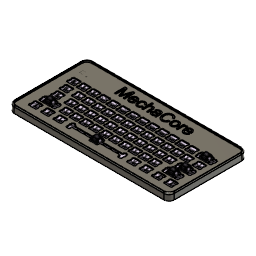
Mechacore (Autodesk Fusion 360 design; units mm, degrees)
description: KiCad electronic assembly
part number: Mechacore 1
part number: D_SOD-123
part number: SW_Cherry_MX_PCB
Autodesk Fusion 360 part; units mm, degrees
(part 1 of 4)
sketch "Sketch1" plane through (0, 0, 0) normal (0, 1, 0) x (1, 0, 0)
  line L0 (0, 0) -> (310, 0)
  line L1 (310, 0) -> (310, 150.9928)
  line L2 (310, 150.9928) -> (0, 150.9928)
  line L3 (0, 150.9928) -> (0, 0)
  dimension "d1" = 310
  constraint horizontal L0
  constraint vertical L1
  constraint horizontal L2
  constraint vertical L3
  constraint coincident L0.start L3.end
  measures "d1" distance of L0.start L0.end
extrude "Extrude1" add sketch "Sketch1" along normal blind 10 makes body 1
extrude "Extrude2" add 1 faces at (206.6667, 10, -50.3309) along direction (0, 1, 0) blind 4 on bodies 1 bodies 1
shell "Shell1" thickness 2 removed faces 1 at (206.6667, 14, -50.3309) on bodies 1
fillet "Fillet1" radius 10 1 edges at (2, 8, -148.9928) on bodies 1
fillet "Fillet2" radius 10 1 edges at (308, 8, -148.9928) on bodies 1
fillet "Fillet3" radius 10 1 edges at (308, 8, -2) on bodies 1
fillet "Fillet4" radius 10 1 edges at (2, 8, -2) on bodies 1
fillet "Fillet5" radius 10 3 edges at (310, 7, -150.9928) (0, 7, -150.9928) (310, 7, 0) on bodies 1
fillet "Fillet6" radius 10 1 edges at (0, 7, 0) on bodies 1
other "Base Mesh Feature1"
other "Modify1"
other "Modify2"
sketch "48cd8e48e3c34c88b59e201f8eb7611360cf066c_switch" plane through (0, 0, 0) normal (0, 1, 0) x (1, 0, 0)
  line L0 (0.0951, 95.5075) -> (285.845, 95.5075)
  line L1 (285.845, 95.5075) -> (285.845, 0.2577)
  line L2 (285.845, 0.2577) -> (0.0951, 0.2577)
  line L3 (0.0951, 0.2577) -> (0.0951, 95.5075)
  line L4 (124.062, 16.7831) -> (124.062, 15.7827)
  line L5 (124.062, 15.7827) -> (123.263, 15.7827)
  line L6 (123.263, 15.7827) -> (123.263, 12.6848)
  line L7 (123.263, 12.6848) -> (124.062, 12.6848)
  line L8 (124.062, 12.6848) -> (124.062, 12.0826)
  line L9 (124.062, 12.0826) -> (84.4381, 12.0826)
  line L10 (84.4381, 12.0826) -> (84.4381, 15.3128)
  line L11 (84.4381, 15.3128) -> (82.7126, 15.3128)
  line L12 (82.7126, 15.3128) -> (82.7126, 16.2347)
  line L13 (82.7126, 16.2347) -> (79.412, 16.2347)
  line L14 (79.412, 16.2347) -> (79.412, 15.3128)
  line L15 (79.412, 15.3128) -> (77.687, 15.3128)
  line L16 (77.687, 15.3128) -> (77.687, 12.0826)
  line L17 (77.687, 12.0826) -> (76.8629, 12.0826)
  line L18 (76.8629, 12.0826) -> (76.8629, 9.2838)
  line L19 (76.8629, 9.2838) -> (77.687, 9.2838)
  line L20 (77.687, 9.2838) -> (77.687, 3.0138)
  line L21 (77.687, 3.0138) -> (79.412, 3.0138)
  line L22 (79.412, 3.0138) -> (79.412, 2.0326)
  line L23 (79.412, 2.0326) -> (82.7126, 2.0326)
  line L24 (82.7126, 2.0326) -> (82.7126, 3.0138)
  line L25 (82.7126, 3.0138) -> (84.4381, 3.0138)
  line L26 (84.4381, 3.0138) -> (84.4381, 7.4841)
  line L27 (84.4381, 7.4841) -> (124.062, 7.4841)
  line L28 (124.062, 7.4841) -> (124.062, 6.8833)
  line L29 (124.062, 6.8833) -> (123.263, 6.8833)
  line L30 (123.263, 6.8833) -> (123.263, 3.7827)
  line L31 (123.263, 3.7827) -> (124.062, 3.7827)
  line L32 (124.062, 3.7827) -> (124.062, 2.7836)
  line L33 (124.062, 2.7836) -> (138.063, 2.7836)
  line L34 (138.063, 2.7836) -> (138.063, 3.7827)
  line L35 (138.063, 3.7827) -> (138.862, 3.7827)
  line L36 (138.862, 3.7827) -> (138.862, 6.8833)
  line L37 (138.862, 6.8833) -> (138.063, 6.8833)
  line L38 (138.063, 6.8833) -> (138.063, 7.4841)
  line L39 (138.063, 7.4841) -> (177.687, 7.4841)
  line L40 (177.687, 7.4841) -> (177.687, 3.0138)
  line L41 (177.687, 3.0138) -> (179.412, 3.0138)
  line L42 (179.412, 3.0138) -> (179.412, 2.0326)
  line L43 (179.412, 2.0326) -> (182.713, 2.0326)
  line L44 (182.713, 2.0326) -> (182.713, 3.0138)
  line L45 (182.713, 3.0138) -> (184.438, 3.0138)
  line L46 (184.438, 3.0138) -> (184.438, 9.2838)
  line L47 (184.438, 9.2838) -> (185.262, 9.2838)
  line L48 (185.262, 9.2838) -> (185.262, 12.0826)
  line L49 (185.262, 12.0826) -> (184.438, 12.0826)
  line L50 (184.438, 12.0826) -> (184.438, 15.3128)
  line L51 (184.438, 15.3128) -> (182.713, 15.3128)
  line L52 (182.713, 15.3128) -> (182.713, 16.2347)
  line L53 (182.713, 16.2347) -> (179.412, 16.2347)
  line L54 (179.412, 16.2347) -> (179.412, 15.3128)
  line L55 (179.412, 15.3128) -> (177.687, 15.3128)
  line L56 (177.687, 15.3128) -> (177.687, 12.0826)
  line L57 (177.687, 12.0826) -> (138.063, 12.0826)
  line L58 (138.063, 12.0826) -> (138.063, 12.6848)
  line L59 (138.063, 12.6848) -> (138.862, 12.6848)
  line L60 (138.862, 12.6848) -> (138.862, 15.7827)
  line L61 (138.862, 15.7827) -> (138.063, 15.7827)
  line L62 (138.063, 15.7827) -> (138.063, 16.7831)
  line L63 (138.063, 16.7831) -> (124.062, 16.7831)
  line L64 (5.0009, 16.7831) -> (5.0009, 15.7827)
  line L65 (5.0009, 15.7827) -> (4.2003, 15.7827)
  line L66 (4.2003, 15.7827) -> (4.2003, 12.6848)
  line L67 (4.2003, 12.6848) -> (5.0009, 12.6848)
  line L68 (5.0009, 12.6848) -> (5.0009, 6.8833)
  line L69 (5.0009, 6.8833) -> (4.2003, 6.8833)
  line L70 (4.2003, 6.8833) -> (4.2003, 3.7827)
  line L71 (4.2003, 3.7827) -> (5.0009, 3.7827)
  line L72 (5.0009, 3.7827) -> (5.0009, 2.7836)
  line L73 (5.0009, 2.7836) -> (19.0004, 2.7836)
  line L74 (19.0004, 2.7836) -> (19.0004, 3.7827)
  line L75 (19.0004, 3.7827) -> (19.801, 3.7827)
  line L76 (19.801, 3.7827) -> (19.801, 6.8833)
  line L77 (19.801, 6.8833) -> (19.0004, 6.8833)
  line L78 (19.0004, 6.8833) -> (19.0004, 12.6848)
  line L79 (19.0004, 12.6848) -> (19.801, 12.6848)
  line L80 (19.801, 12.6848) -> (19.801, 15.7827)
  line L81 (19.801, 15.7827) -> (19.0004, 15.7827)
  line L82 (19.0004, 15.7827) -> (19.0004, 16.7831)
  line L83 (19.0004, 16.7831) -> (5.0009, 16.7831)
  line L84 (28.812, 16.7831) -> (28.812, 15.7827)
  line L85 (28.812, 15.7827) -> (28.0128, 15.7827)
  line L86 (28.0128, 15.7827) -> (28.0128, 12.6848)
  line L87 (28.0128, 12.6848) -> (28.812, 12.6848)
  line L88 (28.812, 12.6848) -> (28.812, 6.8833)
  line L89 (28.812, 6.8833) -> (28.0128, 6.8833)
  line L90 (28.0128, 6.8833) -> (28.0128, 3.7827)
  line L91 (28.0128, 3.7827) -> (28.812, 3.7827)
  line L92 (28.812, 3.7827) -> (28.812, 2.7836)
  line L93 (28.812, 2.7836) -> (42.8128, 2.7836)
  line L94 (42.8128, 2.7836) -> (42.8128, 3.7827)
  line L95 (42.8128, 3.7827) -> (43.6122, 3.7827)
  line L96 (43.6122, 3.7827) -> (43.6122, 6.8833)
  line L97 (43.6122, 6.8833) -> (42.8128, 6.8833)
  line L98 (42.8128, 6.8833) -> (42.8128, 12.6848)
  line L99 (42.8128, 12.6848) -> (43.6122, 12.6848)
  line L100 (43.6122, 12.6848) -> (43.6122, 15.7827)
  line L101 (43.6122, 15.7827) -> (42.8128, 15.7827)
  line L102 (42.8128, 15.7827) -> (42.8128, 16.7831)
  line L103 (42.8128, 16.7831) -> (28.812, 16.7831)
  line L104 (52.626, 16.7831) -> (52.626, 15.7827)
  line L105 (52.626, 15.7827) -> (51.8252, 15.7827)
  line L106 (51.8252, 15.7827) -> (51.8252, 12.6848)
  line L107 (51.8252, 12.6848) -> (52.626, 12.6848)
  line L108 (52.626, 12.6848) -> (52.626, 6.8833)
  line L109 (52.626, 6.8833) -> (51.8252, 6.8833)
  line L110 (51.8252, 6.8833) -> (51.8252, 3.7827)
  line L111 (51.8252, 3.7827) -> (52.626, 3.7827)
  line L112 (52.626, 3.7827) -> (52.626, 2.7836)
  line L113 (52.626, 2.7836) -> (66.6253, 2.7836)
  line L114 (66.6253, 2.7836) -> (66.6253, 3.7827)
  line L115 (66.6253, 3.7827) -> (67.4261, 3.7827)
  line L116 (67.4261, 3.7827) -> (67.4261, 6.8833)
  line L117 (67.4261, 6.8833) -> (66.6253, 6.8833)
  line L118 (66.6253, 6.8833) -> (66.6253, 12.6848)
  line L119 (66.6253, 12.6848) -> (67.4261, 12.6848)
  line L120 (67.4261, 12.6848) -> (67.4261, 15.7827)
  line L121 (67.4261, 15.7827) -> (66.6253, 15.7827)
  line L122 (66.6253, 15.7827) -> (66.6253, 16.7831)
  line L123 (66.6253, 16.7831) -> (52.626, 16.7831)
  line L124 (195.501, 16.7831) -> (195.501, 15.7827)
  line L125 (195.501, 15.7827) -> (194.7, 15.7827)
  line L126 (194.7, 15.7827) -> (194.7, 12.6848)
  line L127 (194.7, 12.6848) -> (195.501, 12.6848)
  line L128 (195.501, 12.6848) -> (195.501, 6.8833)
  line L129 (195.501, 6.8833) -> (194.7, 6.8833)
  line L130 (194.7, 6.8833) -> (194.7, 3.7827)
  line L131 (194.7, 3.7827) -> (195.501, 3.7827)
  line L132 (195.501, 3.7827) -> (195.501, 2.7836)
  line L133 (195.501, 2.7836) -> (209.5, 2.7836)
  line L134 (209.5, 2.7836) -> (209.5, 3.7827)
  line L135 (209.5, 3.7827) -> (210.301, 3.7827)
  line L136 (210.301, 3.7827) -> (210.301, 6.8833)
  line L137 (210.301, 6.8833) -> (209.5, 6.8833)
  line L138 (209.5, 6.8833) -> (209.5, 12.6848)
  line L139 (209.5, 12.6848) -> (210.301, 12.6848)
  line L140 (210.301, 12.6848) -> (210.301, 15.7827)
  line L141 (210.301, 15.7827) -> (209.5, 15.7827)
  line L142 (209.5, 15.7827) -> (209.5, 16.7831)
  line L143 (209.5, 16.7831) -> (195.501, 16.7831)
  line L144 (219.312, 16.7831) -> (219.312, 15.7827)
  line L145 (219.312, 15.7827) -> (218.513, 15.7827)
  line L146 (218.513, 15.7827) -> (218.513, 12.6848)
  line L147 (218.513, 12.6848) -> (219.312, 12.6848)
  line L148 (219.312, 12.6848) -> (219.312, 6.8833)
  line L149 (219.312, 6.8833) -> (218.513, 6.8833)
  line L150 (218.513, 6.8833) -> (218.513, 3.7827)
  line L151 (218.513, 3.7827) -> (219.312, 3.7827)
  line L152 (219.312, 3.7827) -> (219.312, 2.7836)
  line L153 (219.312, 2.7836) -> (233.313, 2.7836)
  line L154 (233.313, 2.7836) -> (233.313, 3.7827)
  line L155 (233.313, 3.7827) -> (234.112, 3.7827)
  line L156 (234.112, 3.7827) -> (234.112, 6.8833)
  line L157 (234.112, 6.8833) -> (233.313, 6.8833)
  line L158 (233.313, 6.8833) -> (233.313, 12.6848)
  line L159 (233.313, 12.6848) -> (234.112, 12.6848)
  line L160 (234.112, 12.6848) -> (234.112, 15.7827)
  line L161 (234.112, 15.7827) -> (233.313, 15.7827)
  line L162 (233.313, 15.7827) -> (233.313, 16.7831)
  line L163 (233.313, 16.7831) -> (219.312, 16.7831)
  line L164 (243.126, 16.7831) -> (243.126, 15.7827)
  line L165 (243.126, 15.7827) -> (242.325, 15.7827)
  line L166 (242.325, 15.7827) -> (242.325, 12.6848)
  line L167 (242.325, 12.6848) -> (243.126, 12.6848)
  line L168 (243.126, 12.6848) -> (243.126, 6.8833)
  line L169 (243.126, 6.8833) -> (242.325, 6.8833)
  line L170 (242.325, 6.8833) -> (242.325, 3.7827)
  line L171 (242.325, 3.7827) -> (243.126, 3.7827)
  line L172 (243.126, 3.7827) -> (243.126, 2.7836)
  line L173 (243.126, 2.7836) -> (257.125, 2.7836)
  line L174 (257.125, 2.7836) -> (257.125, 3.7827)
  line L175 (257.125, 3.7827) -> (257.926, 3.7827)
  line L176 (257.926, 3.7827) -> (257.926, 6.8833)
  line L177 (257.926, 6.8833) -> (257.125, 6.8833)
  line L178 (257.125, 6.8833) -> (257.125, 12.6848)
  line L179 (257.125, 12.6848) -> (257.926, 12.6848)
  line L180 (257.926, 12.6848) -> (257.926, 15.7827)
  line L181 (257.926, 15.7827) -> (257.125, 15.7827)
  line L182 (257.125, 15.7827) -> (257.125, 16.7831)
  line L183 (257.125, 16.7831) -> (243.126, 16.7831)
  line L184 (266.937, 16.7831) -> (266.937, 15.7827)
  line L185 (266.937, 15.7827) -> (266.138, 15.7827)
  line L186 (266.138, 15.7827) -> (266.138, 12.6848)
  line L187 (266.138, 12.6848) -> (266.937, 12.6848)
  line L188 (266.937, 12.6848) -> (266.937, 6.8833)
  line L189 (266.937, 6.8833) -> (266.138, 6.8833)
  line L190 (266.138, 6.8833) -> (266.138, 3.7827)
  line L191 (266.138, 3.7827) -> (266.937, 3.7827)
  line L192 (266.937, 3.7827) -> (266.937, 2.7836)
  line L193 (266.937, 2.7836) -> (280.938, 2.7836)
  line L194 (280.938, 2.7836) -> (280.938, 3.7827)
  line L195 (280.938, 3.7827) -> (281.737, 3.7827)
  line L196 (281.737, 3.7827) -> (281.737, 6.8833)
  line L197 (281.737, 6.8833) -> (280.938, 6.8833)
  line L198 (280.938, 6.8833) -> (280.938, 12.6848)
  line L199 (280.938, 12.6848) -> (281.737, 12.6848)
  line L200 (281.737, 12.6848) -> (281.737, 15.7827)
  line L201 (281.737, 15.7827) -> (280.938, 15.7827)
  line L202 (280.938, 15.7827) -> (280.938, 16.7831)
  line L203 (280.938, 16.7831) -> (266.937, 16.7831)
  line L204 (14.5259, 35.833) -> (14.5259, 34.8327)
  line L205 (14.5259, 34.8327) -> (13.7253, 34.8327)
  line L206 (13.7253, 34.8327) -> (13.7253, 31.7348)
  line L207 (13.7253, 31.7348) -> (14.5259, 31.7348)
  line L208 (14.5259, 31.7348) -> (14.5259, 31.1326)
  line L209 (14.5259, 31.1326) -> (13.0004, 31.1326)
  line L210 (13.0004, 31.1326) -> (13.0004, 34.3628)
  line L211 (13.0004, 34.3628) -> (11.2751, 34.3628)
  line L212 (11.2751, 34.3628) -> (11.2751, 35.2848)
  line L213 (11.2751, 35.2848) -> (7.9761, 35.2848)
  line L214 (7.9761, 35.2848) -> (7.9761, 34.3628)
  line L215 (7.9761, 34.3628) -> (6.2508, 34.3628)
  line L216 (6.2508, 34.3628) -> (6.2508, 31.1326)
  line L217 (6.2508, 31.1326) -> (5.4253, 31.1326)
  line L218 (5.4253, 31.1326) -> (5.4253, 28.3338)
  line L219 (5.4253, 28.3338) -> (6.2508, 28.3338)
  line L220 (6.2508, 28.3338) -> (6.2508, 22.0638)
  line L221 (6.2508, 22.0638) -> (7.9761, 22.0638)
  line L222 (7.9761, 22.0638) -> (7.9761, 21.0826)
  line L223 (7.9761, 21.0826) -> (11.2751, 21.0826)
  line L224 (11.2751, 21.0826) -> (11.2751, 22.0638)
  line L225 (11.2751, 22.0638) -> (13.0004, 22.0638)
  line L226 (13.0004, 22.0638) -> (13.0004, 26.5327)
  line L227 (13.0004, 26.5327) -> (14.5259, 26.5327)
  line L228 (14.5259, 26.5327) -> (14.5259, 25.9333)
  line L229 (14.5259, 25.9333) -> (13.7253, 25.9333)
  line L230 (13.7253, 25.9333) -> (13.7253, 22.8327)
  line L231 (13.7253, 22.8327) -> (14.5259, 22.8327)
  line L232 (14.5259, 22.8327) -> (14.5259, 21.8336)
  line L233 (14.5259, 21.8336) -> (28.5254, 21.8336)
  line L234 (28.5254, 21.8336) -> (28.5254, 22.8327)
  line L235 (28.5254, 22.8327) -> (29.326, 22.8327)
  line L236 (29.326, 22.8327) -> (29.326, 25.9333)
  line L237 (29.326, 25.9333) -> (28.5254, 25.9333)
  line L238 (28.5254, 25.9333) -> (28.5254, 26.5327)
  line L239 (28.5254, 26.5327) -> (30.0509, 26.5327)
  line L240 (30.0509, 26.5327) -> (30.0509, 22.0638)
  line L241 (30.0509, 22.0638) -> (31.7748, 22.0638)
  line L242 (31.7748, 22.0638) -> (31.7748, 21.0826)
  line L243 (31.7748, 21.0826) -> (35.0752, 21.0826)
  line L244 (35.0752, 21.0826) -> (35.0752, 22.0638)
  line L245 (35.0752, 22.0638) -> (36.8004, 22.0638)
  line L246 (36.8004, 22.0638) -> (36.8004, 28.3338)
  line L247 (36.8004, 28.3338) -> (37.6259, 28.3338)
  line L248 (37.6259, 28.3338) -> (37.6259, 31.1326)
  line L249 (37.6259, 31.1326) -> (36.8004, 31.1326)
  line L250 (36.8004, 31.1326) -> (36.8004, 34.3628)
  line L251 (36.8004, 34.3628) -> (35.0752, 34.3628)
  line L252 (35.0752, 34.3628) -> (35.0752, 35.2848)
  line L253 (35.0752, 35.2848) -> (31.7748, 35.2848)
  line L254 (31.7748, 35.2848) -> (31.7748, 34.3628)
  line L255 (31.7748, 34.3628) -> (30.0509, 34.3628)
  line L256 (30.0509, 34.3628) -> (30.0509, 31.1326)
  line L257 (30.0509, 31.1326) -> (28.5254, 31.1326)
  line L258 (28.5254, 31.1326) -> (28.5254, 31.7348)
  line L259 (28.5254, 31.7348) -> (29.326, 31.7348)
  line L260 (29.326, 31.7348) -> (29.326, 34.8327)
  line L261 (29.326, 34.8327) -> (28.5254, 34.8327)
  line L262 (28.5254, 34.8327) -> (28.5254, 35.833)
  line L263 (28.5254, 35.833) -> (14.5259, 35.833)
  line L264 (252.65, 35.833) -> (252.65, 34.8327)
  line L265 (252.65, 34.8327) -> (251.849, 34.8327)
  line L266 (251.849, 34.8327) -> (251.849, 31.7348)
  line L267 (251.849, 31.7348) -> (252.65, 31.7348)
  line L268 (252.65, 31.7348) -> (252.65, 31.1326)
  line L269 (252.65, 31.1326) -> (251.126, 31.1326)
  line L270 (251.126, 31.1326) -> (251.126, 34.3628)
  line L271 (251.126, 34.3628) -> (249.4, 34.3628)
  line L272 (249.4, 34.3628) -> (249.4, 35.2848)
  line L273 (249.4, 35.2848) -> (246.101, 35.2848)
  line L274 (246.101, 35.2848) -> (246.101, 34.3628)
  line L275 (246.101, 34.3628) -> (244.376, 34.3628)
  line L276 (244.376, 34.3628) -> (244.376, 31.1326)
  line L277 (244.376, 31.1326) -> (243.55, 31.1326)
  line L278 (243.55, 31.1326) -> (243.55, 28.3338)
  line L279 (243.55, 28.3338) -> (244.376, 28.3338)
  line L280 (244.376, 28.3338) -> (244.376, 22.0638)
  line L281 (244.376, 22.0638) -> (246.101, 22.0638)
  line L282 (246.101, 22.0638) -> (246.101, 21.0826)
  line L283 (246.101, 21.0826) -> (249.4, 21.0826)
  line L284 (249.4, 21.0826) -> (249.4, 22.0638)
  line L285 (249.4, 22.0638) -> (251.126, 22.0638)
  line L286 (251.126, 22.0638) -> (251.126, 26.5327)
  line L287 (251.126, 26.5327) -> (252.65, 26.5327)
  line L288 (252.65, 26.5327) -> (252.65, 25.9333)
  line L289 (252.65, 25.9333) -> (251.849, 25.9333)
  line L290 (251.849, 25.9333) -> (251.849, 22.8327)
  line L291 (251.849, 22.8327) -> (252.65, 22.8327)
  line L292 (252.65, 22.8327) -> (252.65, 21.8336)
  line L293 (252.65, 21.8336) -> (266.65, 21.8336)
  line L294 (266.65, 21.8336) -> (266.65, 22.8327)
  line L295 (266.65, 22.8327) -> (267.451, 22.8327)
  line L296 (267.451, 22.8327) -> (267.451, 25.9333)
  line L297 (267.451, 25.9333) -> (266.65, 25.9333)
  line L298 (266.65, 25.9333) -> (266.65, 26.5327)
  line L299 (266.65, 26.5327) -> (268.176, 26.5327)
  line L300 (268.176, 26.5327) -> (268.176, 22.0638)
  line L301 (268.176, 22.0638) -> (269.9, 22.0638)
  line L302 (269.9, 22.0638) -> (269.9, 21.0826)
  line L303 (269.9, 21.0826) -> (273.2, 21.0826)
  line L304 (273.2, 21.0826) -> (273.2, 22.0638)
  line L305 (273.2, 22.0638) -> (274.925, 22.0638)
  line L306 (274.925, 22.0638) -> (274.925, 28.3338)
  line L307 (274.925, 28.3338) -> (275.751, 28.3338)
  line L308 (275.751, 28.3338) -> (275.751, 31.1326)
  line L309 (275.751, 31.1326) -> (274.925, 31.1326)
  line L310 (274.925, 31.1326) -> (274.925, 34.3628)
  line L311 (274.925, 34.3628) -> (273.2, 34.3628)
  line L312 (273.2, 34.3628) -> (273.2, 35.2848)
  line L313 (273.2, 35.2848) -> (269.9, 35.2848)
  line L314 (269.9, 35.2848) -> (269.9, 34.3628)
  line L315 (269.9, 34.3628) -> (268.176, 34.3628)
  line L316 (268.176, 34.3628) -> (268.176, 31.1326)
  line L317 (268.176, 31.1326) -> (266.65, 31.1326)
  line L318 (266.65, 31.1326) -> (266.65, 31.7348)
  line L319 (266.65, 31.7348) -> (267.451, 31.7348)
  line L320 (267.451, 31.7348) -> (267.451, 34.8327)
  line L321 (267.451, 34.8327) -> (266.65, 34.8327)
  line L322 (266.65, 34.8327) -> (266.65, 35.833)
  line L323 (266.65, 35.833) -> (252.65, 35.833)
  line L324 (45.4822, 35.833) -> (45.4822, 34.8327)
  line L325 (45.4822, 34.8327) -> (44.6814, 34.8327)
  line L326 (44.6814, 34.8327) -> (44.6814, 31.7348)
  line L327 (44.6814, 31.7348) -> (45.4822, 31.7348)
  line L328 (45.4822, 31.7348) -> (45.4822, 25.9333)
  line L329 (45.4822, 25.9333) -> (44.6814, 25.9333)
  line L330 (44.6814, 25.9333) -> (44.6814, 22.8327)
  line L331 (44.6814, 22.8327) -> (45.4822, 22.8327)
  line L332 (45.4822, 22.8327) -> (45.4822, 21.8336)
  line L333 (45.4822, 21.8336) -> (59.4815, 21.8336)
  line L334 (59.4815, 21.8336) -> (59.4815, 22.8327)
  line L335 (59.4815, 22.8327) -> (60.2809, 22.8327)
  line L336 (60.2809, 22.8327) -> (60.2809, 25.9333)
  line L337 (60.2809, 25.9333) -> (59.4815, 25.9333)
  line L338 (59.4815, 25.9333) -> (59.4815, 31.7348)
  line L339 (59.4815, 31.7348) -> (60.2809, 31.7348)
  line L340 (60.2809, 31.7348) -> (60.2809, 34.8327)
  line L341 (60.2809, 34.8327) -> (59.4815, 34.8327)
  line L342 (59.4815, 34.8327) -> (59.4815, 35.833)
  line L343 (59.4815, 35.833) -> (45.4822, 35.833)
  line L344 (64.5322, 35.833) -> (64.5322, 34.8327)
  line L345 (64.5322, 34.8327) -> (63.7314, 34.8327)
  line L346 (63.7314, 34.8327) -> (63.7314, 31.7348)
  line L347 (63.7314, 31.7348) -> (64.5322, 31.7348)
  line L348 (64.5322, 31.7348) -> (64.5322, 25.9333)
  line L349 (64.5322, 25.9333) -> (63.7314, 25.9333)
  line L350 (63.7314, 25.9333) -> (63.7314, 22.8327)
  line L351 (63.7314, 22.8327) -> (64.5322, 22.8327)
  line L352 (64.5322, 22.8327) -> (64.5322, 21.8336)
  line L353 (64.5322, 21.8336) -> (78.5315, 21.8336)
  line L354 (78.5315, 21.8336) -> (78.5315, 22.8327)
  line L355 (78.5315, 22.8327) -> (79.3309, 22.8327)
  line L356 (79.3309, 22.8327) -> (79.3309, 25.9333)
  line L357 (79.3309, 25.9333) -> (78.5315, 25.9333)
  line L358 (78.5315, 25.9333) -> (78.5315, 31.7348)
  line L359 (78.5315, 31.7348) -> (79.3309, 31.7348)
  line L360 (79.3309, 31.7348) -> (79.3309, 34.8327)
  line L361 (79.3309, 34.8327) -> (78.5315, 34.8327)
  line L362 (78.5315, 34.8327) -> (78.5315, 35.833)
  line L363 (78.5315, 35.833) -> (64.5322, 35.833)
  line L364 (83.5822, 35.833) -> (83.5822, 34.8327)
  line L365 (83.5822, 34.8327) -> (82.7814, 34.8327)
  line L366 (82.7814, 34.8327) -> (82.7814, 31.7348)
  line L367 (82.7814, 31.7348) -> (83.5822, 31.7348)
  line L368 (83.5822, 31.7348) -> (83.5822, 25.9333)
  line L369 (83.5822, 25.9333) -> (82.7814, 25.9333)
  line L370 (82.7814, 25.9333) -> (82.7814, 22.8327)
  line L371 (82.7814, 22.8327) -> (83.5822, 22.8327)
  line L372 (83.5822, 22.8327) -> (83.5822, 21.8336)
  line L373 (83.5822, 21.8336) -> (97.5815, 21.8336)
  line L374 (97.5815, 21.8336) -> (97.5815, 22.8327)
  line L375 (97.5815, 22.8327) -> (98.3809, 22.8327)
  line L376 (98.3809, 22.8327) -> (98.3809, 25.9333)
  line L377 (98.3809, 25.9333) -> (97.5815, 25.9333)
  line L378 (97.5815, 25.9333) -> (97.5815, 31.7348)
  line L379 (97.5815, 31.7348) -> (98.3809, 31.7348)
  line L380 (98.3809, 31.7348) -> (98.3809, 34.8327)
  line L381 (98.3809, 34.8327) -> (97.5815, 34.8327)
  line L382 (97.5815, 34.8327) -> (97.5815, 35.833)
  line L383 (97.5815, 35.833) -> (83.5822, 35.833)
  line L384 (102.632, 35.833) -> (102.632, 34.8327)
  line L385 (102.632, 34.8327) -> (101.831, 34.8327)
  line L386 (101.831, 34.8327) -> (101.831, 31.7348)
  line L387 (101.831, 31.7348) -> (102.632, 31.7348)
  line L388 (102.632, 31.7348) -> (102.632, 25.9333)
  line L389 (102.632, 25.9333) -> (101.831, 25.9333)
  line L390 (101.831, 25.9333) -> (101.831, 22.8327)
  line L391 (101.831, 22.8327) -> (102.632, 22.8327)
  line L392 (102.632, 22.8327) -> (102.632, 21.8336)
  line L393 (102.632, 21.8336) -> (116.632, 21.8336)
  line L394 (116.632, 21.8336) -> (116.632, 22.8327)
  line L395 (116.632, 22.8327) -> (117.431, 22.8327)
  line L396 (117.431, 22.8327) -> (117.431, 25.9333)
  line L397 (117.431, 25.9333) -> (116.632, 25.9333)
  line L398 (116.632, 25.9333) -> (116.632, 31.7348)
  line L399 (116.632, 31.7348) -> (117.431, 31.7348)
  line L400 (117.431, 31.7348) -> (117.431, 34.8327)
  line L401 (117.431, 34.8327) -> (116.632, 34.8327)
  line L402 (116.632, 34.8327) -> (116.632, 35.833)
  line L403 (116.632, 35.833) -> (102.632, 35.833)
  line L404 (121.682, 35.833) -> (121.682, 34.8327)
  line L405 (121.682, 34.8327) -> (120.881, 34.8327)
  line L406 (120.881, 34.8327) -> (120.881, 31.7348)
  line L407 (120.881, 31.7348) -> (121.682, 31.7348)
  line L408 (121.682, 31.7348) -> (121.682, 25.9333)
  line L409 (121.682, 25.9333) -> (120.881, 25.9333)
  line L410 (120.881, 25.9333) -> (120.881, 22.8327)
  line L411 (120.881, 22.8327) -> (121.682, 22.8327)
  line L412 (121.682, 22.8327) -> (121.682, 21.8336)
  line L413 (121.682, 21.8336) -> (135.682, 21.8336)
  line L414 (135.682, 21.8336) -> (135.682, 22.8327)
  line L415 (135.682, 22.8327) -> (136.481, 22.8327)
  line L416 (136.481, 22.8327) -> (136.481, 25.9333)
  line L417 (136.481, 25.9333) -> (135.682, 25.9333)
  line L418 (135.682, 25.9333) -> (135.682, 31.7348)
  line L419 (135.682, 31.7348) -> (136.481, 31.7348)
  line L420 (136.481, 31.7348) -> (136.481, 34.8327)
  line L421 (136.481, 34.8327) -> (135.682, 34.8327)
  line L422 (135.682, 34.8327) -> (135.682, 35.833)
  line L423 (135.682, 35.833) -> (121.682, 35.833)
  line L424 (140.732, 35.833) -> (140.732, 34.8327)
  line L425 (140.732, 34.8327) -> (139.931, 34.8327)
  line L426 (139.931, 34.8327) -> (139.931, 31.7348)
  line L427 (139.931, 31.7348) -> (140.732, 31.7348)
  line L428 (140.732, 31.7348) -> (140.732, 25.9333)
  line L429 (140.732, 25.9333) -> (139.931, 25.9333)
  line L430 (139.931, 25.9333) -> (139.931, 22.8327)
  line L431 (139.931, 22.8327) -> (140.732, 22.8327)
  line L432 (140.732, 22.8327) -> (140.732, 21.8336)
  line L433 (140.732, 21.8336) -> (154.732, 21.8336)
  line L434 (154.732, 21.8336) -> (154.732, 22.8327)
  line L435 (154.732, 22.8327) -> (155.531, 22.8327)
  line L436 (155.531, 22.8327) -> (155.531, 25.9333)
  line L437 (155.531, 25.9333) -> (154.732, 25.9333)
  line L438 (154.732, 25.9333) -> (154.732, 31.7348)
  line L439 (154.732, 31.7348) -> (155.531, 31.7348)
  line L440 (155.531, 31.7348) -> (155.531, 34.8327)
  line L441 (155.531, 34.8327) -> (154.732, 34.8327)
  line L442 (154.732, 34.8327) -> (154.732, 35.833)
  line L443 (154.732, 35.833) -> (140.732, 35.833)
  line L444 (159.782, 35.833) -> (159.782, 34.8327)
  line L445 (159.782, 34.8327) -> (158.981, 34.8327)
  line L446 (158.981, 34.8327) -> (158.981, 31.7348)
  line L447 (158.981, 31.7348) -> (159.782, 31.7348)
  line L448 (159.782, 31.7348) -> (159.782, 25.9333)
  line L449 (159.782, 25.9333) -> (158.981, 25.9333)
  line L450 (158.981, 25.9333) -> (158.981, 22.8327)
  line L451 (158.981, 22.8327) -> (159.782, 22.8327)
  line L452 (159.782, 22.8327) -> (159.782, 21.8336)
  line L453 (159.782, 21.8336) -> (173.782, 21.8336)
  line L454 (173.782, 21.8336) -> (173.782, 22.8327)
  line L455 (173.782, 22.8327) -> (174.581, 22.8327)
  line L456 (174.581, 22.8327) -> (174.581, 25.9333)
  line L457 (174.581, 25.9333) -> (173.782, 25.9333)
  line L458 (173.782, 25.9333) -> (173.782, 31.7348)
  line L459 (173.782, 31.7348) -> (174.581, 31.7348)
  line L460 (174.581, 31.7348) -> (174.581, 34.8327)
  line L461 (174.581, 34.8327) -> (173.782, 34.8327)
  line L462 (173.782, 34.8327) -> (173.782, 35.833)
  line L463 (173.782, 35.833) -> (159.782, 35.833)
  line L464 (178.832, 35.833) -> (178.832, 34.8327)
  line L465 (178.832, 34.8327) -> (178.031, 34.8327)
  line L466 (178.031, 34.8327) -> (178.031, 31.7348)
  line L467 (178.031, 31.7348) -> (178.832, 31.7348)
  line L468 (178.832, 31.7348) -> (178.832, 25.9333)
  line L469 (178.832, 25.9333) -> (178.031, 25.9333)
  line L470 (178.031, 25.9333) -> (178.031, 22.8327)
  line L471 (178.031, 22.8327) -> (178.832, 22.8327)
  line L472 (178.832, 22.8327) -> (178.832, 21.8336)
  line L473 (178.832, 21.8336) -> (192.832, 21.8336)
  line L474 (192.832, 21.8336) -> (192.832, 22.8327)
  line L475 (192.832, 22.8327) -> (193.631, 22.8327)
  line L476 (193.631, 22.8327) -> (193.631, 25.9333)
  line L477 (193.631, 25.9333) -> (192.832, 25.9333)
  line L478 (192.832, 25.9333) -> (192.832, 31.7348)
  line L479 (192.832, 31.7348) -> (193.631, 31.7348)
  line L480 (193.631, 31.7348) -> (193.631, 34.8327)
  line L481 (193.631, 34.8327) -> (192.832, 34.8327)
  line L482 (192.832, 34.8327) -> (192.832, 35.833)
  line L483 (192.832, 35.833) -> (178.832, 35.833)
  line L484 (197.882, 35.833) -> (197.882, 34.8327)
  line L485 (197.882, 34.8327) -> (197.081, 34.8327)
  line L486 (197.081, 34.8327) -> (197.081, 31.7348)
  line L487 (197.081, 31.7348) -> (197.882, 31.7348)
  line L488 (197.882, 31.7348) -> (197.882, 25.9333)
  line L489 (197.882, 25.9333) -> (197.081, 25.9333)
  line L490 (197.081, 25.9333) -> (197.081, 22.8327)
  line L491 (197.081, 22.8327) -> (197.882, 22.8327)
  line L492 (197.882, 22.8327) -> (197.882, 21.8336)
  line L493 (197.882, 21.8336) -> (211.882, 21.8336)
  line L494 (211.882, 21.8336) -> (211.882, 22.8327)
  line L495 (211.882, 22.8327) -> (212.681, 22.8327)
  line L496 (212.681, 22.8327) -> (212.681, 25.9333)
  line L497 (212.681, 25.9333) -> (211.882, 25.9333)
  line L498 (211.882, 25.9333) -> (211.882, 31.7348)
  line L499 (211.882, 31.7348) -> (212.681, 31.7348)
  line L500 (212.681, 31.7348) -> (212.681, 34.8327)
  line L501 (212.681, 34.8327) -> (211.882, 34.8327)
  line L502 (211.882, 34.8327) -> (211.882, 35.833)
  line L503 (211.882, 35.833) -> (197.882, 35.833)
  line L504 (216.932, 35.833) -> (216.932, 34.8327)
  line L505 (216.932, 34.8327) -> (216.131, 34.8327)
  line L506 (216.131, 34.8327) -> (216.131, 31.7348)
  line L507 (216.131, 31.7348) -> (216.932, 31.7348)
  line L508 (216.932, 31.7348) -> (216.932, 25.9333)
  line L509 (216.932, 25.9333) -> (216.131, 25.9333)
  line L510 (216.131, 25.9333) -> (216.131, 22.8327)
  line L511 (216.131, 22.8327) -> (216.932, 22.8327)
  line L512 (216.932, 22.8327) -> (216.932, 21.8336)
  line L513 (216.932, 21.8336) -> (230.932, 21.8336)
  line L514 (230.932, 21.8336) -> (230.932, 22.8327)
  line L515 (230.932, 22.8327) -> (231.731, 22.8327)
  line L516 (231.731, 22.8327) -> (231.731, 25.9333)
  line L517 (231.731, 25.9333) -> (230.932, 25.9333)
  line L518 (230.932, 25.9333) -> (230.932, 31.7348)
  line L519 (230.932, 31.7348) -> (231.731, 31.7348)
  line L520 (231.731, 31.7348) -> (231.731, 34.8327)
  line L521 (231.731, 34.8327) -> (230.932, 34.8327)
  line L522 (230.932, 34.8327) -> (230.932, 35.833)
  line L523 (230.932, 35.833) -> (216.932, 35.833)
  line L524 (257.412, 54.8831) -> (257.412, 53.8826)
  line L525 (257.412, 53.8826) -> (256.611, 53.8826)
  line L526 (256.611, 53.8826) -> (256.611, 50.7834)
  line L527 (256.611, 50.7834) -> (257.412, 50.7834)
  line L528 (257.412, 50.7834) -> (257.412, 50.1826)
  line L529 (257.412, 50.1826) -> (255.888, 50.1826)
  line L530 (255.888, 50.1826) -> (255.888, 53.4127)
  line L531 (255.888, 53.4127) -> (254.161, 53.4127)
  line L532 (254.161, 53.4127) -> (254.161, 54.3334)
  line L533 (254.161, 54.3334) -> (250.862, 54.3334)
  line L534 (250.862, 54.3334) -> (250.862, 53.4127)
  line L535 (250.862, 53.4127) -> (249.137, 53.4127)
  line L536 (249.137, 53.4127) -> (249.137, 50.1826)
  line L537 (249.137, 50.1826) -> (248.313, 50.1826)
  line L538 (248.313, 50.1826) -> (248.313, 47.3837)
  line L539 (248.313, 47.3837) -> (249.137, 47.3837)
  line L540 (249.137, 47.3837) -> (249.137, 41.1138)
  line L541 (249.137, 41.1138) -> (250.862, 41.1138)
  line L542 (250.862, 41.1138) -> (250.862, 40.1327)
  line L543 (250.862, 40.1327) -> (254.161, 40.1327)
  line L544 (254.161, 40.1327) -> (254.161, 41.1138)
  line L545 (254.161, 41.1138) -> (255.888, 41.1138)
  line L546 (255.888, 41.1138) -> (255.888, 45.5828)
  line L547 (255.888, 45.5828) -> (257.412, 45.5828)
  line L548 (257.412, 45.5828) -> (257.412, 44.9834)
  line L549 (257.412, 44.9834) -> (256.611, 44.9834)
  line L550 (256.611, 44.9834) -> (256.611, 41.8828)
  line L551 (256.611, 41.8828) -> (257.412, 41.8828)
  line L552 (257.412, 41.8828) -> (257.412, 40.8838)
  line L553 (257.412, 40.8838) -> (271.413, 40.8838)
  line L554 (271.413, 40.8838) -> (271.413, 41.8828)
  line L555 (271.413, 41.8828) -> (272.212, 41.8828)
  line L556 (272.212, 41.8828) -> (272.212, 44.9834)
  line L557 (272.212, 44.9834) -> (271.413, 44.9834)
  line L558 (271.413, 44.9834) -> (271.413, 45.5828)
  line L559 (271.413, 45.5828) -> (272.937, 45.5828)
  line L560 (272.937, 45.5828) -> (272.937, 41.1138)
  line L561 (272.937, 41.1138) -> (274.662, 41.1138)
  line L562 (274.662, 41.1138) -> (274.662, 40.1327)
  line L563 (274.662, 40.1327) -> (277.963, 40.1327)
  line L564 (277.963, 40.1327) -> (277.963, 41.1138)
  line L565 (277.963, 41.1138) -> (279.688, 41.1138)
  line L566 (279.688, 41.1138) -> (279.688, 47.3837)
  line L567 (279.688, 47.3837) -> (280.512, 47.3837)
  line L568 (280.512, 47.3837) -> (280.512, 50.1826)
  line L569 (280.512, 50.1826) -> (279.688, 50.1826)
  line L570 (279.688, 50.1826) -> (279.688, 53.4127)
  line L571 (279.688, 53.4127) -> (277.963, 53.4127)
  line L572 (277.963, 53.4127) -> (277.963, 54.3334)
  line L573 (277.963, 54.3334) -> (274.662, 54.3334)
  line L574 (274.662, 54.3334) -> (274.662, 53.4127)
  line L575 (274.662, 53.4127) -> (272.937, 53.4127)
  line L576 (272.937, 53.4127) -> (272.937, 50.1826)
  line L577 (272.937, 50.1826) -> (271.413, 50.1826)
  line L578 (271.413, 50.1826) -> (271.413, 50.7834)
  line L579 (271.413, 50.7834) -> (272.212, 50.7834)
  line L580 (272.212, 50.7834) -> (272.212, 53.8826)
  line L581 (272.212, 53.8826) -> (271.413, 53.8826)
  line L582 (271.413, 53.8826) -> (271.413, 54.8831)
  line L583 (271.413, 54.8831) -> (257.412, 54.8831)
  line L584 (9.762, 54.8831) -> (9.762, 53.8826)
  line L585 (9.762, 53.8826) -> (8.9628, 53.8826)
  line L586 (8.9628, 53.8826) -> (8.9628, 50.7834)
  line L587 (8.9628, 50.7834) -> (9.762, 50.7834)
  line L588 (9.762, 50.7834) -> (9.762, 44.9834)
  line L589 (9.762, 44.9834) -> (8.9628, 44.9834)
  line L590 (8.9628, 44.9834) -> (8.9628, 41.8828)
  line L591 (8.9628, 41.8828) -> (9.762, 41.8828)
  line L592 (9.762, 41.8828) -> (9.762, 40.8838)
  line L593 (9.762, 40.8838) -> (23.7629, 40.8838)
  line L594 (23.7629, 40.8838) -> (23.7629, 41.8828)
  line L595 (23.7629, 41.8828) -> (24.5622, 41.8828)
  line L596 (24.5622, 41.8828) -> (24.5622, 44.9834)
  line L597 (24.5622, 44.9834) -> (23.7629, 44.9834)
  line L598 (23.7629, 44.9834) -> (23.7629, 50.7834)
  line L599 (23.7629, 50.7834) -> (24.5622, 50.7834)
  line L600 (24.5622, 50.7834) -> (24.5622, 53.8826)
  line L601 (24.5622, 53.8826) -> (23.7629, 53.8826)
  line L602 (23.7629, 53.8826) -> (23.7629, 54.8831)
  line L603 (23.7629, 54.8831) -> (9.762, 54.8831)
  line L604 (35.9572, 54.8831) -> (35.9572, 53.8826)
  line L605 (35.9572, 53.8826) -> (35.1565, 53.8826)
  line L606 (35.1565, 53.8826) -> (35.1565, 50.7834)
  line L607 (35.1565, 50.7834) -> (35.9572, 50.7834)
  line L608 (35.9572, 50.7834) -> (35.9572, 44.9834)
  line L609 (35.9572, 44.9834) -> (35.1565, 44.9834)
  line L610 (35.1565, 44.9834) -> (35.1565, 41.8828)
  line L611 (35.1565, 41.8828) -> (35.9572, 41.8828)
  line L612 (35.9572, 41.8828) -> (35.9572, 40.8838)
  line L613 (35.9572, 40.8838) -> (49.9565, 40.8838)
  line L614 (49.9565, 40.8838) -> (49.9565, 41.8828)
  line L615 (49.9565, 41.8828) -> (50.7559, 41.8828)
  line L616 (50.7559, 41.8828) -> (50.7559, 44.9834)
  line L617 (50.7559, 44.9834) -> (49.9565, 44.9834)
  line L618 (49.9565, 44.9834) -> (49.9565, 50.7834)
  line L619 (49.9565, 50.7834) -> (50.7559, 50.7834)
  line L620 (50.7559, 50.7834) -> (50.7559, 53.8826)
  line L621 (50.7559, 53.8826) -> (49.9565, 53.8826)
  line L622 (49.9565, 53.8826) -> (49.9565, 54.8831)
  line L623 (49.9565, 54.8831) -> (35.9572, 54.8831)
  line L624 (55.0072, 54.8831) -> (55.0072, 53.8826)
  line L625 (55.0072, 53.8826) -> (54.2064, 53.8826)
  line L626 (54.2064, 53.8826) -> (54.2064, 50.7834)
  line L627 (54.2064, 50.7834) -> (55.0072, 50.7834)
  line L628 (55.0072, 50.7834) -> (55.0072, 44.9834)
  line L629 (55.0072, 44.9834) -> (54.2064, 44.9834)
  line L630 (54.2064, 44.9834) -> (54.2064, 41.8828)
  line L631 (54.2064, 41.8828) -> (55.0072, 41.8828)
  line L632 (55.0072, 41.8828) -> (55.0072, 40.8838)
  line L633 (55.0072, 40.8838) -> (69.0065, 40.8838)
  line L634 (69.0065, 40.8838) -> (69.0065, 41.8828)
  line L635 (69.0065, 41.8828) -> (69.8059, 41.8828)
  line L636 (69.8059, 41.8828) -> (69.8059, 44.9834)
  line L637 (69.8059, 44.9834) -> (69.0065, 44.9834)
  line L638 (69.0065, 44.9834) -> (69.0065, 50.7834)
  line L639 (69.0065, 50.7834) -> (69.8059, 50.7834)
  line L640 (69.8059, 50.7834) -> (69.8059, 53.8826)
  line L641 (69.8059, 53.8826) -> (69.0065, 53.8826)
  line L642 (69.0065, 53.8826) -> (69.0065, 54.8831)
  line L643 (69.0065, 54.8831) -> (55.0072, 54.8831)
  line L644 (74.0572, 54.8831) -> (74.0572, 53.8826)
  line L645 (74.0572, 53.8826) -> (73.2564, 53.8826)
  line L646 (73.2564, 53.8826) -> (73.2564, 50.7834)
  line L647 (73.2564, 50.7834) -> (74.0572, 50.7834)
  line L648 (74.0572, 50.7834) -> (74.0572, 44.9834)
  line L649 (74.0572, 44.9834) -> (73.2564, 44.9834)
  line L650 (73.2564, 44.9834) -> (73.2564, 41.8828)
  line L651 (73.2564, 41.8828) -> (74.0572, 41.8828)
  line L652 (74.0572, 41.8828) -> (74.0572, 40.8838)
  line L653 (74.0572, 40.8838) -> (88.0565, 40.8838)
  line L654 (88.0565, 40.8838) -> (88.0565, 41.8828)
  line L655 (88.0565, 41.8828) -> (88.8559, 41.8828)
  line L656 (88.8559, 41.8828) -> (88.8559, 44.9834)
  line L657 (88.8559, 44.9834) -> (88.0565, 44.9834)
  line L658 (88.0565, 44.9834) -> (88.0565, 50.7834)
  line L659 (88.0565, 50.7834) -> (88.8559, 50.7834)
  line L660 (88.8559, 50.7834) -> (88.8559, 53.8826)
  line L661 (88.8559, 53.8826) -> (88.0565, 53.8826)
  line L662 (88.0565, 53.8826) -> (88.0565, 54.8831)
  line L663 (88.0565, 54.8831) -> (74.0572, 54.8831)
  line L664 (93.1072, 54.8831) -> (93.1072, 53.8826)
  line L665 (93.1072, 53.8826) -> (92.3064, 53.8826)
  line L666 (92.3064, 53.8826) -> (92.3064, 50.7834)
  line L667 (92.3064, 50.7834) -> (93.1072, 50.7834)
  line L668 (93.1072, 50.7834) -> (93.1072, 44.9834)
  line L669 (93.1072, 44.9834) -> (92.3064, 44.9834)
  line L670 (92.3064, 44.9834) -> (92.3064, 41.8828)
  line L671 (92.3064, 41.8828) -> (93.1072, 41.8828)
  line L672 (93.1072, 41.8828) -> (93.1072, 40.8838)
  line L673 (93.1072, 40.8838) -> (107.107, 40.8838)
  line L674 (107.107, 40.8838) -> (107.107, 41.8828)
  line L675 (107.107, 41.8828) -> (107.906, 41.8828)
  line L676 (107.906, 41.8828) -> (107.906, 44.9834)
  line L677 (107.906, 44.9834) -> (107.107, 44.9834)
  line L678 (107.107, 44.9834) -> (107.107, 50.7834)
  line L679 (107.107, 50.7834) -> (107.906, 50.7834)
  line L680 (107.906, 50.7834) -> (107.906, 53.8826)
  line L681 (107.906, 53.8826) -> (107.107, 53.8826)
  line L682 (107.107, 53.8826) -> (107.107, 54.8831)
  line L683 (107.107, 54.8831) -> (93.1072, 54.8831)
  line L684 (112.157, 54.8831) -> (112.157, 53.8826)
  line L685 (112.157, 53.8826) -> (111.356, 53.8826)
  line L686 (111.356, 53.8826) -> (111.356, 50.7834)
  line L687 (111.356, 50.7834) -> (112.157, 50.7834)
  line L688 (112.157, 50.7834) -> (112.157, 44.9834)
  line L689 (112.157, 44.9834) -> (111.356, 44.9834)
  line L690 (111.356, 44.9834) -> (111.356, 41.8828)
  line L691 (111.356, 41.8828) -> (112.157, 41.8828)
  line L692 (112.157, 41.8828) -> (112.157, 40.8838)
  line L693 (112.157, 40.8838) -> (126.157, 40.8838)
  line L694 (126.157, 40.8838) -> (126.157, 41.8828)
  line L695 (126.157, 41.8828) -> (126.956, 41.8828)
  line L696 (126.956, 41.8828) -> (126.956, 44.9834)
  line L697 (126.956, 44.9834) -> (126.157, 44.9834)
  line L698 (126.157, 44.9834) -> (126.157, 50.7834)
  line L699 (126.157, 50.7834) -> (126.956, 50.7834)
  line L700 (126.956, 50.7834) -> (126.956, 53.8826)
  line L701 (126.956, 53.8826) -> (126.157, 53.8826)
  line L702 (126.157, 53.8826) -> (126.157, 54.8831)
  line L703 (126.157, 54.8831) -> (112.157, 54.8831)
  line L704 (131.207, 54.8831) -> (131.207, 53.8826)
  line L705 (131.207, 53.8826) -> (130.406, 53.8826)
  line L706 (130.406, 53.8826) -> (130.406, 50.7834)
  line L707 (130.406, 50.7834) -> (131.207, 50.7834)
  line L708 (131.207, 50.7834) -> (131.207, 44.9834)
  line L709 (131.207, 44.9834) -> (130.406, 44.9834)
  line L710 (130.406, 44.9834) -> (130.406, 41.8828)
  line L711 (130.406, 41.8828) -> (131.207, 41.8828)
  line L712 (131.207, 41.8828) -> (131.207, 40.8838)
  line L713 (131.207, 40.8838) -> (145.207, 40.8838)
  line L714 (145.207, 40.8838) -> (145.207, 41.8828)
  line L715 (145.207, 41.8828) -> (146.006, 41.8828)
  line L716 (146.006, 41.8828) -> (146.006, 44.9834)
  line L717 (146.006, 44.9834) -> (145.207, 44.9834)
  line L718 (145.207, 44.9834) -> (145.207, 50.7834)
  line L719 (145.207, 50.7834) -> (146.006, 50.7834)
  line L720 (146.006, 50.7834) -> (146.006, 53.8826)
  line L721 (146.006, 53.8826) -> (145.207, 53.8826)
  line L722 (145.207, 53.8826) -> (145.207, 54.8831)
  line L723 (145.207, 54.8831) -> (131.207, 54.8831)
  line L724 (150.257, 54.8831) -> (150.257, 53.8826)
  line L725 (150.257, 53.8826) -> (149.456, 53.8826)
  line L726 (149.456, 53.8826) -> (149.456, 50.7834)
  line L727 (149.456, 50.7834) -> (150.257, 50.7834)
  line L728 (150.257, 50.7834) -> (150.257, 44.9834)
  line L729 (150.257, 44.9834) -> (149.456, 44.9834)
  line L730 (149.456, 44.9834) -> (149.456, 41.8828)
  line L731 (149.456, 41.8828) -> (150.257, 41.8828)
  line L732 (150.257, 41.8828) -> (150.257, 40.8838)
  line L733 (150.257, 40.8838) -> (164.257, 40.8838)
  line L734 (164.257, 40.8838) -> (164.257, 41.8828)
  line L735 (164.257, 41.8828) -> (165.056, 41.8828)
  line L736 (165.056, 41.8828) -> (165.056, 44.9834)
  line L737 (165.056, 44.9834) -> (164.257, 44.9834)
  line L738 (164.257, 44.9834) -> (164.257, 50.7834)
  line L739 (164.257, 50.7834) -> (165.056, 50.7834)
  line L740 (165.056, 50.7834) -> (165.056, 53.8826)
  line L741 (165.056, 53.8826) -> (164.257, 53.8826)
  line L742 (164.257, 53.8826) -> (164.257, 54.8831)
  line L743 (164.257, 54.8831) -> (150.257, 54.8831)
  line L744 (169.307, 54.8831) -> (169.307, 53.8826)
  line L745 (169.307, 53.8826) -> (168.506, 53.8826)
  line L746 (168.506, 53.8826) -> (168.506, 50.7834)
  line L747 (168.506, 50.7834) -> (169.307, 50.7834)
  line L748 (169.307, 50.7834) -> (169.307, 44.9834)
  line L749 (169.307, 44.9834) -> (168.506, 44.9834)
  line L750 (168.506, 44.9834) -> (168.506, 41.8828)
  line L751 (168.506, 41.8828) -> (169.307, 41.8828)
  line L752 (169.307, 41.8828) -> (169.307, 40.8838)
  line L753 (169.307, 40.8838) -> (183.307, 40.8838)
  line L754 (183.307, 40.8838) -> (183.307, 41.8828)
  line L755 (183.307, 41.8828) -> (184.106, 41.8828)
  line L756 (184.106, 41.8828) -> (184.106, 44.9834)
  line L757 (184.106, 44.9834) -> (183.307, 44.9834)
  line L758 (183.307, 44.9834) -> (183.307, 50.7834)
  line L759 (183.307, 50.7834) -> (184.106, 50.7834)
  line L760 (184.106, 50.7834) -> (184.106, 53.8826)
  line L761 (184.106, 53.8826) -> (183.307, 53.8826)
  line L762 (183.307, 53.8826) -> (183.307, 54.8831)
  line L763 (183.307, 54.8831) -> (169.307, 54.8831)
  line L764 (188.357, 54.8831) -> (188.357, 53.8826)
  line L765 (188.357, 53.8826) -> (187.556, 53.8826)
  line L766 (187.556, 53.8826) -> (187.556, 50.7834)
  line L767 (187.556, 50.7834) -> (188.357, 50.7834)
  line L768 (188.357, 50.7834) -> (188.357, 44.9834)
  line L769 (188.357, 44.9834) -> (187.556, 44.9834)
  line L770 (187.556, 44.9834) -> (187.556, 41.8828)
  line L771 (187.556, 41.8828) -> (188.357, 41.8828)
  line L772 (188.357, 41.8828) -> (188.357, 40.8838)
  line L773 (188.357, 40.8838) -> (202.357, 40.8838)
  line L774 (202.357, 40.8838) -> (202.357, 41.8828)
  line L775 (202.357, 41.8828) -> (203.156, 41.8828)
  line L776 (203.156, 41.8828) -> (203.156, 44.9834)
  line L777 (203.156, 44.9834) -> (202.357, 44.9834)
  line L778 (202.357, 44.9834) -> (202.357, 50.7834)
  line L779 (202.357, 50.7834) -> (203.156, 50.7834)
  line L780 (203.156, 50.7834) -> (203.156, 53.8826)
  line L781 (203.156, 53.8826) -> (202.357, 53.8826)
  line L782 (202.357, 53.8826) -> (202.357, 54.8831)
  line L783 (202.357, 54.8831) -> (188.357, 54.8831)
  line L784 (207.407, 54.8831) -> (207.407, 53.8826)
  line L785 (207.407, 53.8826) -> (206.606, 53.8826)
  line L786 (206.606, 53.8826) -> (206.606, 50.7834)
  line L787 (206.606, 50.7834) -> (207.407, 50.7834)
  line L788 (207.407, 50.7834) -> (207.407, 44.9834)
  line L789 (207.407, 44.9834) -> (206.606, 44.9834)
  line L790 (206.606, 44.9834) -> (206.606, 41.8828)
  line L791 (206.606, 41.8828) -> (207.407, 41.8828)
  line L792 (207.407, 41.8828) -> (207.407, 40.8838)
  line L793 (207.407, 40.8838) -> (221.407, 40.8838)
  line L794 (221.407, 40.8838) -> (221.407, 41.8828)
  line L795 (221.407, 41.8828) -> (222.206, 41.8828)
  line L796 (222.206, 41.8828) -> (222.206, 44.9834)
  line L797 (222.206, 44.9834) -> (221.407, 44.9834)
  line L798 (221.407, 44.9834) -> (221.407, 50.7834)
  line L799 (221.407, 50.7834) -> (222.206, 50.7834)
  line L800 (222.206, 50.7834) -> (222.206, 53.8826)
  line L801 (222.206, 53.8826) -> (221.407, 53.8826)
  line L802 (221.407, 53.8826) -> (221.407, 54.8831)
  line L803 (221.407, 54.8831) -> (207.407, 54.8831)
  line L804 (226.457, 54.8831) -> (226.457, 53.8826)
  line L805 (226.457, 53.8826) -> (225.656, 53.8826)
  line L806 (225.656, 53.8826) -> (225.656, 50.7834)
  line L807 (225.656, 50.7834) -> (226.457, 50.7834)
  line L808 (226.457, 50.7834) -> (226.457, 44.9834)
  line L809 (226.457, 44.9834) -> (225.656, 44.9834)
  line L810 (225.656, 44.9834) -> (225.656, 41.8828)
  line L811 (225.656, 41.8828) -> (226.457, 41.8828)
  line L812 (226.457, 41.8828) -> (226.457, 40.8838)
  line L813 (226.457, 40.8838) -> (240.457, 40.8838)
  line L814 (240.457, 40.8838) -> (240.457, 41.8828)
  line L815 (240.457, 41.8828) -> (241.256, 41.8828)
  line L816 (241.256, 41.8828) -> (241.256, 44.9834)
  line L817 (241.256, 44.9834) -> (240.457, 44.9834)
  line L818 (240.457, 44.9834) -> (240.457, 50.7834)
  line L819 (240.457, 50.7834) -> (241.256, 50.7834)
  line L820 (241.256, 50.7834) -> (241.256, 53.8826)
  line L821 (241.256, 53.8826) -> (240.457, 53.8826)
  line L822 (240.457, 53.8826) -> (240.457, 54.8831)
  line L823 (240.457, 54.8831) -> (226.457, 54.8831)
  line L824 (7.3822, 73.9331) -> (7.3822, 72.9326)
  line L825 (7.3822, 72.9326) -> (6.5815, 72.9326)
  line L826 (6.5815, 72.9326) -> (6.5815, 69.8334)
  line L827 (6.5815, 69.8334) -> (7.3822, 69.8334)
  line L828 (7.3822, 69.8334) -> (7.3822, 64.0334)
  line L829 (7.3822, 64.0334) -> (6.5815, 64.0334)
  line L830 (6.5815, 64.0334) -> (6.5815, 60.9328)
  line L831 (6.5815, 60.9328) -> (7.3822, 60.9328)
  line L832 (7.3822, 60.9328) -> (7.3822, 59.9338)
  line L833 (7.3822, 59.9338) -> (21.3817, 59.9338)
  line L834 (21.3817, 59.9338) -> (21.3817, 60.9328)
  line L835 (21.3817, 60.9328) -> (22.1809, 60.9328)
  line L836 (22.1809, 60.9328) -> (22.1809, 64.0334)
  line L837 (22.1809, 64.0334) -> (21.3817, 64.0334)
  line L838 (21.3817, 64.0334) -> (21.3817, 69.8334)
  line L839 (21.3817, 69.8334) -> (22.1809, 69.8334)
  line L840 (22.1809, 69.8334) -> (22.1809, 72.9326)
  line L841 (22.1809, 72.9326) -> (21.3817, 72.9326)
  line L842 (21.3817, 72.9326) -> (21.3817, 73.9331)
  line L843 (21.3817, 73.9331) -> (7.3822, 73.9331)
  line L844 (31.1947, 73.9331) -> (31.1947, 72.9326)
  line L845 (31.1947, 72.9326) -> (30.394, 72.9326)
  line L846 (30.394, 72.9326) -> (30.394, 69.8334)
  line L847 (30.394, 69.8334) -> (31.1947, 69.8334)
  line L848 (31.1947, 69.8334) -> (31.1947, 64.0334)
  line L849 (31.1947, 64.0334) -> (30.394, 64.0334)
  line L850 (30.394, 64.0334) -> (30.394, 60.9328)
  line L851 (30.394, 60.9328) -> (31.1947, 60.9328)
  line L852 (31.1947, 60.9328) -> (31.1947, 59.9338)
  line L853 (31.1947, 59.9338) -> (45.194, 59.9338)
  line L854 (45.194, 59.9338) -> (45.194, 60.9328)
  line L855 (45.194, 60.9328) -> (45.9948, 60.9328)
  line L856 (45.9948, 60.9328) -> (45.9948, 64.0334)
  line L857 (45.9948, 64.0334) -> (45.194, 64.0334)
  line L858 (45.194, 64.0334) -> (45.194, 69.8334)
  line L859 (45.194, 69.8334) -> (45.9948, 69.8334)
  line L860 (45.9948, 69.8334) -> (45.9948, 72.9326)
  line L861 (45.9948, 72.9326) -> (45.194, 72.9326)
  line L862 (45.194, 72.9326) -> (45.194, 73.9331)
  line L863 (45.194, 73.9331) -> (31.1947, 73.9331)
  line L864 (50.2447, 73.9331) -> (50.2447, 72.9326)
  line L865 (50.2447, 72.9326) -> (49.4439, 72.9326)
  line L866 (49.4439, 72.9326) -> (49.4439, 69.8334)
  line L867 (49.4439, 69.8334) -> (50.2447, 69.8334)
  line L868 (50.2447, 69.8334) -> (50.2447, 64.0334)
  line L869 (50.2447, 64.0334) -> (49.4439, 64.0334)
  line L870 (49.4439, 64.0334) -> (49.4439, 60.9328)
  line L871 (49.4439, 60.9328) -> (50.2447, 60.9328)
  line L872 (50.2447, 60.9328) -> (50.2447, 59.9338)
  line L873 (50.2447, 59.9338) -> (64.244, 59.9338)
  line L874 (64.244, 59.9338) -> (64.244, 60.9328)
  line L875 (64.244, 60.9328) -> (65.0448, 60.9328)
  line L876 (65.0448, 60.9328) -> (65.0448, 64.0334)
  line L877 (65.0448, 64.0334) -> (64.244, 64.0334)
  line L878 (64.244, 64.0334) -> (64.244, 69.8334)
  line L879 (64.244, 69.8334) -> (65.0448, 69.8334)
  line L880 (65.0448, 69.8334) -> (65.0448, 72.9326)
  line L881 (65.0448, 72.9326) -> (64.244, 72.9326)
  line L882 (64.244, 72.9326) -> (64.244, 73.9331)
  line L883 (64.244, 73.9331) -> (50.2447, 73.9331)
  line L884 (69.2947, 73.9331) -> (69.2947, 72.9326)
  line L885 (69.2947, 72.9326) -> (68.4939, 72.9326)
  line L886 (68.4939, 72.9326) -> (68.4939, 69.8334)
  line L887 (68.4939, 69.8334) -> (69.2947, 69.8334)
  line L888 (69.2947, 69.8334) -> (69.2947, 64.0334)
  line L889 (69.2947, 64.0334) -> (68.4939, 64.0334)
  line L890 (68.4939, 64.0334) -> (68.4939, 60.9328)
  line L891 (68.4939, 60.9328) -> (69.2947, 60.9328)
  line L892 (69.2947, 60.9328) -> (69.2947, 59.9338)
  line L893 (69.2947, 59.9338) -> (83.294, 59.9338)
  line L894 (83.294, 59.9338) -> (83.294, 60.9328)
  line L895 (83.294, 60.9328) -> (84.0948, 60.9328)
  line L896 (84.0948, 60.9328) -> (84.0948, 64.0334)
  line L897 (84.0948, 64.0334) -> (83.294, 64.0334)
  line L898 (83.294, 64.0334) -> (83.294, 69.8334)
  line L899 (83.294, 69.8334) -> (84.0948, 69.8334)
  line L900 (84.0948, 69.8334) -> (84.0948, 72.9326)
  line L901 (84.0948, 72.9326) -> (83.294, 72.9326)
  line L902 (83.294, 72.9326) -> (83.294, 73.9331)
  line L903 (83.294, 73.9331) -> (69.2947, 73.9331)
  line L904 (88.3447, 73.9331) -> (88.3447, 72.9326)
  line L905 (88.3447, 72.9326) -> (87.5439, 72.9326)
  line L906 (87.5439, 72.9326) -> (87.5439, 69.8334)
  line L907 (87.5439, 69.8334) -> (88.3447, 69.8334)
  line L908 (88.3447, 69.8334) -> (88.3447, 64.0334)
  line L909 (88.3447, 64.0334) -> (87.5439, 64.0334)
  line L910 (87.5439, 64.0334) -> (87.5439, 60.9328)
  line L911 (87.5439, 60.9328) -> (88.3447, 60.9328)
  line L912 (88.3447, 60.9328) -> (88.3447, 59.9338)
  line L913 (88.3447, 59.9338) -> (102.344, 59.9338)
  line L914 (102.344, 59.9338) -> (102.344, 60.9328)
  line L915 (102.344, 60.9328) -> (103.145, 60.9328)
  line L916 (103.145, 60.9328) -> (103.145, 64.0334)
  line L917 (103.145, 64.0334) -> (102.344, 64.0334)
  line L918 (102.344, 64.0334) -> (102.344, 69.8334)
  line L919 (102.344, 69.8334) -> (103.145, 69.8334)
  line L920 (103.145, 69.8334) -> (103.145, 72.9326)
  line L921 (103.145, 72.9326) -> (102.344, 72.9326)
  line L922 (102.344, 72.9326) -> (102.344, 73.9331)
  line L923 (102.344, 73.9331) -> (88.3447, 73.9331)
  line L924 (107.395, 73.9331) -> (107.395, 72.9326)
  line L925 (107.395, 72.9326) -> (106.594, 72.9326)